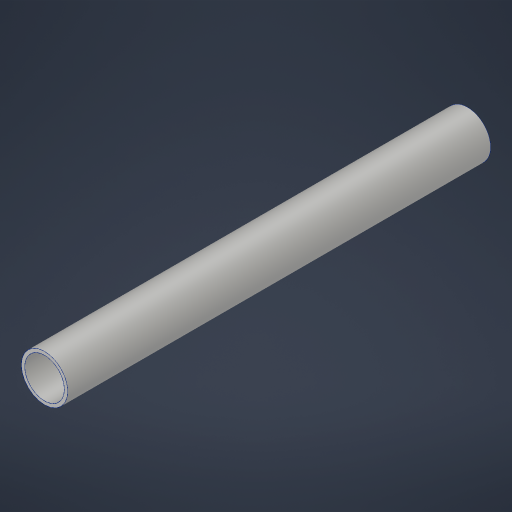
# Autodesk Inventor part: EL2-C-004
Saved by Autodesk Inventor 2023.4 (Build 274418000, 418)
## iProperties
Created: 2025-01-11
Part Number: EL2-C-004
Material: Aluminum 6061
Document SubType Name: Modeling
Designer: brand
Density: 2.7 g/cm^3
Appearance: Aluminum - Flat
Author: brand
Autodesk Inventor part; units mm, degrees
ref_plane "YZ Plane" through (0, 0, 0) normal (1, 0, 0) x (0, 1, 0)
ref_plane "XZ Plane" through (0, 0, 0) normal (0, 1, 0) x (-1, 0, 0)
ref_plane "XY Plane" through (0, 0, 0) normal (0, 0, 1) x (1, 0, 0)
sketch "Sketch1" plane through (0, 0, 0) normal (0, 0, 1) x (1, 0, 0)
  circle A0 centre (0, 0) radius 11.1125
  circle A1 centre (0, 0) radius 9.525
  dimension "d0" = 22.225
  dimension "d1" = 1.5875
  constraints: 2 centre point, 1 coincident
  measures "d0" diameter of A0
  measures "d1" radial gap between concentric circles of A0 A1
extrude "Extrusion1" add sketch "Sketch1" along normal mid plane 203.2
body "Solid1"
